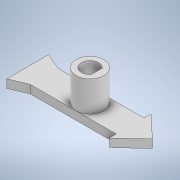
# Autodesk Inventor part: Motor_arrow_v02
Saved by Autodesk Inventor 2022 (Build 260153000, 153)
## iProperties
Created: 2022-07-20
Part Number: Motor_arrow_v02
Material: Generic
Document SubType Name: Modeling
Designer: Bruno
Density: 1 g/cm^3
Appearance: Default
Author: Bruno
Autodesk Inventor part; units mm, degrees
ref_plane "YZ Plane" through (0, 0, 0) normal (1, 0, 0) x (0, 1, 0)
ref_plane "XZ Plane" through (0, 0, 0) normal (0, 1, 0) x (-1, 0, 0)
ref_plane "XY Plane" through (0, 0, 0) normal (0, 0, 1) x (1, 0, 0)
sketch "Sketch1" plane through (0, 0, 0) normal (0, 1, 0) x (-1, 0, 0)
  line L0 (22.5, -7.5) -> (22.5, 7.5)
  line L1 (22.5, 7.5) -> (-22.5, 7.5)
  line L2 (-22.5, -7.5) -> (22.5, -7.5)
  line L3 (-30, 0) -> (22.5, 0)
  line L4 (-22.5, -7.5) -> (-22.5, 7.5)
  line L5 (0, -7.5) -> (0, 7.5)
  line L6 (-22.5, -7.5) -> (-22.5, 7.5)
  point P0 (0, 0)
  dimension "d0" = 15
  dimension "d1" = 45
  constraints: 14 end point, 4 midpoint, 2 equal length, 2 vertical, 1 horizontal, 1 perpendicular, 1 point on line
  measures "d0" distance of L0.start L0.end
  measures "d1" distance of L2.start L0.start
extrude "Extrusion1" add sketch "Sketch1" along normal blind 3
sketch "Sketch2" plane through (0, 3, 0) normal (0, 1, 0) x (1, 0, 0)
  circle A0 centre (0, 0) radius 5
  arc A1 (2.4, 1.9621) -> (2.4, -1.9621) centre (0, 0) ccw
  line L0 (2.4, 1.9621) -> (2.4, -1.9621)
  dimension "d4" = 10
  dimension "d5" = 3.1
  dimension "d6" = 2.4
  constraints: 2 centre point, 2 coincident, 2 end point, 2 point on circle, 1 vertical
  measures "d4" diameter of A0
  measures "d5" radius of A1
  measures "d6" distance from line of point (0, 0) L0
extrude "Extrusion2" add sketch "Sketch2" along normal blind 11
sketch "Sketch3" plane through (0, 3, 0) normal (0, 1, 0) x (1, 0, 0)
  line L0 (22.5, -7.5) -> (22.5, 7.5) projected
  line L1 (22.5, 0) -> (14.5, 7.5)
  line L2 (22.5, 7.5) -> (-22.5, 7.5) projected
  line L3 (14.5, 7.5) -> (14.5, 5)
  line L4 (14.5, 5) -> (-16.5, 5)
  line L5 (-22.5, 7.5) -> (-22.5, -7.5) projected
  line L6 (-16.5, 5) -> (-22.5, 7.5)
  line L7 (-22.5, 7.5) -> (-22.5, -7.5)
  line L8 (-22.5, 0) -> (22.5, 0)
  line L9 (22.5, 0) -> (14.5, -7.5)
  line L10 (-22.5, -7.5) -> (22.5, -7.5) projected
  line L11 (14.5, -7.5) -> (14.5, -5)
  line L12 (14.5, -5) -> (-16.5, -5)
  line L13 (-16.5, -5) -> (-22.5, -7.5)
  point P0 (0, 0)
  dimension "d9" = 2.5
  dimension "d10" = 8
  dimension "d11" = 6
  dimension "d14" = 6
  dimension "d15" = 2.5
  dimension "d16" = 8
  constraints: 20 end point, 4 perpendicular, 2 midpoint, 2 point on line, 1 collinear, 1 vertical
  measures "d9" distance of L1.end L3.end
  measures "d10" distance between parallel lines of L0 L3
  measures "d11" distance from line of L5 L4.end
  measures "d14" distance from line of L5 L12.end
  measures "d15" distance of L9.end L11.end
  measures "d16" distance between parallel lines of L0 L11
extrude "Extrusion3" cut sketch "Sketch3" against normal through all contours L10 L9 L0 | L1 L2 L0 | L10 L13 L12 L11 | L3 L4 L6 L2
body "Solid1"
